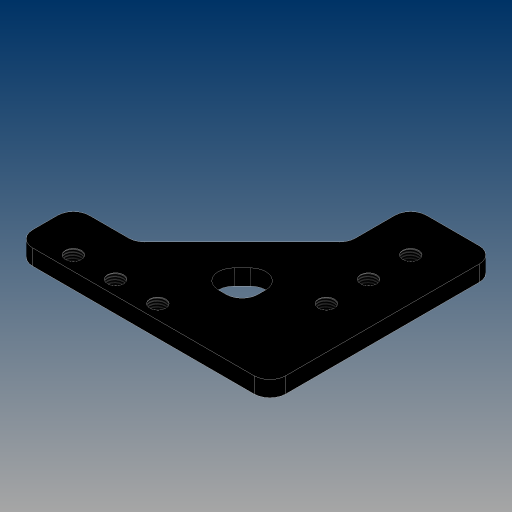
# Autodesk Inventor part: ELEV_012_SUPBRK2_THRD
Saved by Autodesk Inventor 2024.3 (Build 283343000, 343)
## iProperties
Created: 2024-11-26
Part Number: ELEV_012_SUPBRK2_THRD
Material: Aluminum 6061
Document SubType Name: Modeling
Designer: Kenji
Density: 2.7 g/cm^3
Appearance: Anodized - Black
Author: Kenji
Autodesk Inventor part; units mm, degrees
ref_plane "YZ Plane" through (0, 0, 0) normal (1, 0, 0) x (0, 1, 0)
ref_plane "XZ Plane" through (0, 0, 0) normal (0, 1, 0) x (-1, 0, 0)
ref_plane "XY Plane" through (0, 0, 0) normal (0, 0, 1) x (1, 0, 0)
sketch "Sketch1" plane through (0, 0, 0) normal (0, 1, 0) x (-1, 0, 0)
  line L0 (0, -4.7625) -> (0, -64.3255)
  line L1 (4.7625, -69.088) -> (20.6375, -69.088)
  line L2 (76.2, -13.5255) -> (76.2, -4.7625)
  line L3 (71.4375, 0) -> (4.7625, 0)
  circle A0 centre (12.7, -30.988) radius 2.413
  arc A1 (4.7625, 0) -> (0, -4.7625) centre (4.7625, -4.7625) ccw
  circle A2 centre (12.7, -43.688) radius 2.413
  circle A3 centre (12.7, -56.388) radius 2.413
  circle A4 centre (38.1, -5.588) radius 2.413
  circle A5 centre (50.8, -5.588) radius 2.413
  circle A6 centre (63.5, -5.588) radius 2.413
  line L4 (14.4062, -54.6818) -> (61.7938, -7.2942) construction
  line L5 (26.7949, -49.0283) -> (56.1403, -19.6829)
  line L6 (33.5301, -28.8227) -> (35.9347, -26.4181)
  line L7 (25.4, -69.088) -> (25.4, -18.288) construction
  line L8 (76.2, -18.288) -> (25.4, -18.288) construction
  line L9 (25.4, -52.3959) -> (25.4, -64.3255)
  line L10 (71.4375, -18.288) -> (59.5079, -18.288)
  arc A7 (71.4375, -18.288) -> (76.2, -13.5255) centre (71.4375, -13.5255) ccw
  arc A8 (76.2, -4.7625) -> (71.4375, 0) centre (71.4375, -4.7625) ccw
  arc A9 (20.6375, -69.088) -> (25.4, -64.3255) centre (20.6375, -64.3255) ccw
  arc A10 (0, -64.3255) -> (4.7625, -69.088) centre (4.7625, -64.3255) ccw
  line L11 (32.5671, -18.288) -> (30.1625, -18.288)
  line L12 (25.4, -25.4551) -> (25.4, -23.0505)
  arc A11 (59.5079, -18.288) -> (56.1403, -19.6829) centre (59.5079, -23.0505) ccw
  arc A12 (26.7949, -49.0283) -> (25.4, -52.3959) centre (30.1625, -52.3959) ccw
  arc A13 (35.9347, -26.4181) -> (32.5671, -18.288) centre (32.5671, -23.0505) ccw
  arc A14 (25.4, -25.4551) -> (33.5301, -28.8227) centre (30.1625, -25.4551) ccw
  arc A15 (30.1625, -18.288) -> (25.4, -23.0505) centre (30.1625, -23.0505) ccw
  point P0 (0, 0)
  point P1 (0, 7.112)
  point P2 (0, -69.088)
  point P3 (25.4, -50.4232)
  point P4 (57.5352, -18.288)
  point P5 (25.4, -36.9528)
  point P6 (44.0648, -18.288)
  dimension "d0" = 76.2
  dimension "d1" = 4.826
  dimension "d2" = 4.7625
  dimension "d3" = 12.7
  dimension "d4" = 12.7
  dimension "d5" = 12.7
  dimension "d7" = 12.7
  dimension "d8" = 12.7
  dimension "d9" = 38.1
  dimension "d10" = 25.4
  dimension "d11" = 4.7625
  dimension "d12" = 4.7625
  dimension "d13" = 4.7625
  dimension "d14" = 4.7625
  dimension "d15" = 4.7625
  dimension "d16" = 18.288
  dimension "d17" = 25.4
  dimension "d18" = 76.2
  dimension "d19" = 12.7
  dimension "d20" = 38.1
  constraints: 26 end point, 25 point on line, 20 point on circle, 20 tangent, 14 centre point, 7 equal radius, 3 perpendicular, 3 vertical, 2 horizontal, 2 horizontal alignment, 2 parallel, 2 vertical alignment, 1 collinear, 10 other
  measures "d0" distance between parallel lines of L0 L2
  measures "d1" diameter of A0
  measures "d2" radius of A1
  measures "d3" distance from line of L0 point (12.7, -56.388)
  measures "d4" distance of A2.centre A0.centre
  measures "d5" distance of point (12.7, -56.388) A2.centre
  measures "d7" distance of A4.centre A5.centre
  measures "d8" distance of A5.centre point (63.5, -5.588)
  measures "d9" distance from line of L0 A4.centre
  measures "d10" distance of point (0, -69.088) L7.start
  measures "d11" distance between parallel lines of L4 L5
  measures "d12" distance between parallel lines of L4 L6
  measures "d13" radius of A7
  measures "d14" radius of A9
  measures "d15" radius of A11
  measures "d16" distance between parallel lines of L3 L10
  measures "d17" distance from line of point (0, 7.112) L8
  measures "d18" distance from line of point (0, 7.112) L1
  measures "d19" vertical distance of point (0, 7.112) A4.centre
  measures "d20" vertical distance of point (0, 7.112) A0.centre
extrude "Extrusion1" add sketch "Sketch1" along normal blind 4.7625
thread "Thread2" size "10-32 UNF" class "2B" standard "ANSI Unified Screw Threads" full length
thread "Thread3" size "10-32 UNF" class "2B" standard "ANSI Unified Screw Threads" full length
thread "Thread4" size "10-32 UNF" class "2B" standard "ANSI Unified Screw Threads" full length
thread "Thread5" size "10-32 UNF" class "2B" standard "ANSI Unified Screw Threads" full length
thread "Thread6" size "10-32 UNF" class "2B" standard "ANSI Unified Screw Threads" full length
thread "Thread7" size "10-32 UNF" class "2B" standard "ANSI Unified Screw Threads" full length
sketch "Sketch2" plane through (0, 4.7625, 0) normal (0, 1, 0) x (1, 0, 0)
  line L0 (-71.4375, 0) -> (-4.7625, 0) projected
  line L1 (-76.2, 1.27) -> (0, 1.27)
  line L2 (-76.2, 13.5255) -> (-76.2, 4.7625) projected
  line L3 (0, 4.7625) -> (0, 64.3255) projected
  line L4 (0, 1.27) -> (0, 0)
  line L5 (0, 0) -> (-76.2, 0)
  line L6 (-76.2, 0) -> (-76.2, 1.27)
  dimension "d37" = 1.27
  constraints: 8 end point, 2 perpendicular, 2 point on line, 1 parallel, 1 vertical
  measures "d37" distance between parallel lines of L0 L1
extrude "Extrusion2" cut sketch "Sketch2" against normal through all
fillet "Fillet1" radius 4.7752 2 edges at (-74.6754, 2.3813, -1.27) (-1.5246, 2.3813, -1.27)
body "Solid1"
